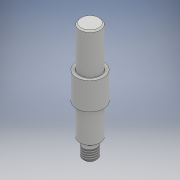
# Autodesk Inventor part: 3강 축1
Saved by Autodesk Inventor 2018.3 (Build 223284000, 284)
## iProperties
Created: 2019-10-11
Part Number: 3강 축1
Material: 일반
Document SubType Name: Modeling
Designer: MyTool
Density: 1 g/cm^3
Appearance: 기본값
Author: MyTool
Autodesk Inventor part; units mm, degrees
ref_plane "YZ Plane" through (0, 0, 0) normal (1, 0, 0) x (0, 1, 0)
ref_plane "XZ Plane" through (0, 0, 0) normal (0, 1, 0) x (-1, 0, 0)
ref_plane "XY Plane" through (0, 0, 0) normal (0, 0, 1) x (1, 0, 0)
sketch "스케치1" plane through (0, 0, 0) normal (1, 0, 0) x (0, 1, 0)
  line L0 (0, 0) -> (5, 0)
  line L1 (5, 0) -> (5, 13)
  line L2 (5, 13) -> (0, 13)
  line L3 (0, 13) -> (0, 0)
  line L4 (0, 13) -> (7.5, 13)
  line L5 (7.5, 13) -> (7.5, 36)
  line L6 (7.5, 36) -> (0, 36)
  line L7 (0, 36) -> (0, 13)
  line L8 (0, 36) -> (10, 36)
  line L9 (10, 36) -> (10, 56)
  line L10 (10, 56) -> (0, 56)
  line L11 (0, 56) -> (0, 36)
  line L12 (0, 56) -> (7.5, 56)
  line L13 (7.5, 56) -> (7.5, 86)
  line L14 (7.5, 86) -> (0, 86)
  line L15 (0, 86) -> (0, 56)
  dimension "d0" = 10
  dimension "d1" = 15
  dimension "d2" = 20
  dimension "d3" = 15
  dimension "d4" = 13
  dimension "d5" = 23
  dimension "d6" = 20
  dimension "d7" = 30
  constraints: 32 end point, 8 parallel, 4 horizontal, 4 perpendicular
  measures "d0" diameter of L1 L3
  measures "d1" diameter of L5 L7
  measures "d2" diameter of L9 L11
  measures "d3" diameter of L13 L15
  measures "d4" distance between parallel lines of L2 L0
  measures "d5" distance of L4.end L5.end
  measures "d6" distance between parallel lines of L10 L6
  measures "d7" distance between parallel lines of L14 L12
revolve "회전1" add sketch "스케치1" angle 360 about axis through (0, 0, 36) along (0, 0, -1)
sketch "스케치2" plane through (0, 0, 0) normal (1, 0, 0) x (0, 1, 0)
  line L0 (5, 8.5) -> (5, 13)
  line L1 (5, 13) -> (3.85, 13)
  line L2 (3.85, 13) -> (3.85, 10.5)
  line L3 (3.85, 10.5) -> (5, 8.5)
  line L4 (-5, 13) -> (5, 13) projected
  line L5 (0, -17.2) -> (0, 103.2) projected
  point P0 (0, 0)
  dimension "d9" = 4.5
  dimension "d10" = 1.15
  dimension "d11" = 2.5
  constraints: 8 end point, 2 perpendicular, 1 vertical
  measures "d9" distance of L0.end L0.start
  measures "d10" distance of L0.end L1.end
  measures "d11" distance of L1.end L2.end
revolve "회전3" cut sketch "스케치2" angle 360 about axis through (0, 0, -10) along (0, 0, 1)
fillet "모깎기1" radius 0.8 2 edges at (0, -3.85, 10.5) (0, -3.85, 13)
thread "스레드1" size "M10x1.5" class "6g" standard "ANSI Metric M Profile" full length
chamfer "모따기1" distance 1 angle 45 2 edges at (0, -5, 0) (0, -7.5, 86)
sketch "스케치3" plane through (0, 0, 0) normal (1, 0, 0) x (0, 1, 0)
  line L0 (11.8435, 67) -> (4.5, 67)
  line L1 (4.5, 67) -> (4.5, 82)
  line L2 (4.5, 82) -> (11.8435, 82)
  line L3 (11.8435, 82) -> (11.8435, 67)
  line L4 (-7.5, 86) -> (7.5, 86) projected
  line L5 (7.5, 86) -> (7.5, 56) projected
  point P0 (0, 0)
  dimension "d20" = 15
  dimension "d21" = 4
  dimension "d22" = 3
  constraints: 8 end point, 2 parallel, 1 horizontal, 1 perpendicular
  measures "d20" distance of L2.end L0.start
  measures "d21" distance between parallel lines of L2 L4
  measures "d22" distance between parallel lines of L5 L1
extrude "돌출1" cut sketch "스케치3" along normal mid plane 5
fillet "모깎기2" radius 2.5 4 edges at (2.5, 5.7855, 67) (-2.5, 5.7855, 67) (-2.5, 5.7855, 82) (2.5, 5.7855, 82)
fillet "모깎기3" radius 0.3 2 edges at (0, -7.5, 36) (0, -7.5, 56)
